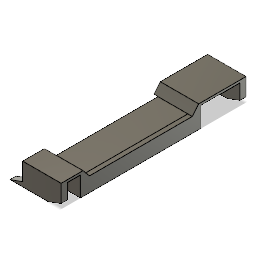
Key v5 (Autodesk Fusion 360 design; units mm, degrees)
Autodesk Fusion 360 part; units mm, degrees
sketch "Sketch1" plane through (0, 0, 0) normal (0, 1, 0) x (1, 0, 0)
  line L0 (15, 72) -> (-15, 72)
  line L1 (-15, 72) -> (-15, -72)
  line L2 (-15, -72) -> (15, -72)
  line L3 (15, -72) -> (15, 72)
  line L4 (15, 72) -> (-15, -72) construction
  line L5 (-15, 72) -> (15, -72) construction
  dimension "d1" = 30
  dimension "d4" = 144
extrude "Extrude1" add sketch "Sketch1" along normal blind 17.5
sketch "Sketch2" plane through (15, 0, 0) normal (1, 0, 0) x (0, 0, -1)
  line L0 (-72, 0) -> (72, 0)
  line L1 (72, 0) -> (72, 17.5)
  line L2 (72, 17.5) -> (-72, 17.5)
  line L3 (-72, 17.5) -> (-72, 0)
  line L4 (-67, 0) -> (-57, 0)
  line L5 (-57, 0) -> (-57, 15.6)
  line L6 (-57, 15.6) -> (-67, 15.6)
  line L7 (-67, 15.6) -> (-67, 0)
  line L8 (67, 0) -> (37, 0)
  line L9 (37, 0) -> (37, 15.6)
  line L10 (37, 15.6) -> (67, 15.6)
  line L11 (67, 15.6) -> (67, 0)
  dimension "d5" = 10
  dimension "d6" = 5
  dimension "d7" = 15.6
  dimension "d8" = 30
  dimension "d9" = 5
  measures "d6" distance of L3 L7
  measures "d7" distance of origin
  measures "d9" distance of L1 L11
extrude "Extrude2" cut sketch "Sketch2" against normal through all contours L0 L4 L5 L6 L7 | L0 L8 L9 L10 L11
sketch "Sketch3" plane through (-15, 0, 0) normal (-1, 0, 0) x (0, 0, 1)
  line L0 (67, 15.6) -> (67, 0)
  line L1 (67, 0) -> (72, 0)
  line L2 (72, 0) -> (72, 17.5)
  line L3 (72, 17.5) -> (-72, 17.5)
  line L4 (-72, 17.5) -> (-72, 0)
  line L5 (-72, 0) -> (-67, 0)
  line L6 (-67, 0) -> (-67, 15.6)
  line L7 (-67, 15.6) -> (-37, 15.6)
  line L8 (-37, 15.6) -> (-37, 0)
  line L9 (-37, 0) -> (57, 0)
  line L10 (57, 0) -> (57, 15.6)
  line L11 (57, 15.6) -> (67, 15.6)
  line L12 (-37, 0) -> (53, 0)
  line L13 (53, 0) -> (53, 7)
  line L14 (53, 7) -> (-37, 7)
  line L15 (-37, 7) -> (-37, 0)
  dimension "d11" = 7
  dimension "d12" = 4
  measures "d11" distance of origin
  measures "d12" distance of L10 L13
extrude "Extrude3" cut sketch "Sketch3" against normal blind 26.5 contours L8 L9 L12 L13 L14 L15
sketch "Sketch4" plane through (-15, 0, 0) normal (-1, 0, 0) x (0, 0, 1)
  line L0 (53, 7) -> (53, 0)
  line L1 (53, 0) -> (57, 0)
  line L2 (57, 0) -> (57, 15.6)
  line L3 (57, 15.6) -> (67, 15.6)
  line L4 (67, 15.6) -> (67, 0)
  line L5 (67, 0) -> (72, 0)
  line L6 (72, 0) -> (72, 17.5)
  line L7 (72, 17.5) -> (-72, 17.5)
  line L8 (-72, 17.5) -> (-72, 0)
  line L9 (-72, 0) -> (-67, 0)
  line L10 (-67, 0) -> (-67, 15.6)
  line L11 (-67, 15.6) -> (-37, 15.6)
  line L12 (-37, 15.6) -> (-37, 7)
  line L13 (-37, 7) -> (53, 7)
  line L14 (-35, 17.5) -> (-30, 11.5)
  line L15 (-30, 11.5) -> (50, 11.5)
  line L16 (50, 11.5) -> (55, 17.5)
  dimension "d15" = 37
  dimension "d16" = 6
  dimension "d17" = 7
  dimension "d18" = 17
  dimension "d19" = 22
  measures "d17" distance of L12
  measures "d19" distance of L6
extrude "Extrude4" cut sketch "Sketch4" against normal through all contours L7 L14 L15 L16
sketch "Sketch5" plane through (-15, 0, 0) normal (-1, 0, 0) x (0, 0, 1)
  line L0 (55, 17.5) -> (50, 11.5)
  line L1 (50, 11.5) -> (-30, 11.5)
  line L2 (-30, 11.5) -> (-35, 17.5)
  line L3 (-35, 17.5) -> (-72, 17.5)
  line L4 (-72, 17.5) -> (-72, 0)
  line L5 (-72, 0) -> (-67, 0)
  line L6 (-67, 0) -> (-67, 15.6)
  line L7 (-67, 15.6) -> (-37, 15.6)
  line L8 (-37, 15.6) -> (-37, 7)
  line L9 (-37, 7) -> (53, 7)
  line L10 (53, 7) -> (53, 0)
  line L11 (53, 0) -> (57, 0)
  line L12 (57, 0) -> (57, 15.6)
  line L13 (57, 15.6) -> (67, 15.6)
  line L14 (67, 15.6) -> (67, 0)
  line L15 (67, 0) -> (72, 0)
  line L16 (72, 0) -> (72, 17.5)
  line L17 (72, 17.5) -> (55, 17.5)
  line L18 (-35, 11.5) -> (55, 11.5)
  line L19 (55, 11.5) -> (55, 8.3)
  line L20 (55, 8.3) -> (-35, 8.3)
  line L21 (-35, 8.3) -> (-35, 11.5)
  dimension "d21" = 5
  dimension "d22" = 3.2
  dimension "d23" = 5
  measures "d21" distance of L21
  measures "d23" distance of L19
extrude "Extrude5" cut sketch "Sketch5" against normal blind 26.5 contours L1 L18 L19 L20 L21
ref_plane "WorkPlane1" through (0, 8.75, 0) normal (0, 0, -1) x (-1, 0, 0)
sketch "Sketch6" plane through (0, 0, -72) normal (0, 0, -1) x (-1, 0, 0)
  line L0 (-15, 0) -> (15, 0)
  line L1 (15, 0) -> (15, 17.5)
  line L2 (15, 17.5) -> (-15, 17.5)
  line L3 (-15, 17.5) -> (-15, 0)
  line L4 (15, 0) -> (25, 0)
  line L5 (25, 0) -> (15, 3.7)
  dimension "d26" = 3.7
  dimension "d27" = 10
  measures "d27" distance of origin
sketch "Sketch7" plane through (0, 0, -72) normal (0, 0, -1) x (-1, 0, 0)
  line L0 (15, 0) -> (-15, 0)
  line L1 (-15, 0) -> (-5, 0)
  line L2 (-15, 0) -> (-15, 17.5)
  line L3 (-5, 0) -> (-15, 3.7)
  line L4 (-15, 0) -> (-15, 3.7)
  dimension "d28" = 10
  dimension "d29" = 3.7
extrude "Extrude6" add sketch "Sketch6" against normal up to surface (5 mm away) contours L1 L4 L5
extrude "Extrude7" cut sketch "Sketch7" against normal up to surface (5 mm away)
mirror "Mirror1" about plane through (0, 8.75, 0) normal (0, 0, -1) of "Extrude6", "Extrude7"
sketch "Sketch8" plane through (0, 0, -72) normal (0, 0, -1) x (-1, 0, 0)
  line L0 (-15, 3.7) -> (-5, 0)
  line L1 (-5, 0) -> (25, 0)
  line L2 (25, 0) -> (15, 3.7)
  line L3 (15, 3.7) -> (15, 17.5)
  line L4 (15, 17.5) -> (-15, 17.5)
  line L5 (-15, 17.5) -> (-15, 3.7)
  circle A0 centre (1.75, 10) radius 2.5
  line L6 (-11.5, 7) -> (15, 7) construction
  line L7 (1.75, 10) -> (1.75, 7) construction
  dimension "d35" = 5
  dimension "d36" = 5
  measures "d35" diameter of A0
  measures "d36" distance of L4 A0
extrude "Extrude8" cut sketch "Sketch8" against normal up to surface (5 mm away) contours A0
sketch "Sketch9" plane through (0, 0, 57) normal (0, 0, 1) x (1, 0, 0)
  line L0 (-15, 15.6) -> (-15, 0)
  line L1 (-15, 0) -> (15, 0)
  line L2 (15, 0) -> (15, 15.6)
  line L3 (15, 15.6) -> (-15, 15.6)
  line L4 (1.25, 12.5) -> (-4.75, 12.5)
  line L5 (-4.75, 12.5) -> (-4.75, 6.5)
  line L6 (-4.75, 6.5) -> (1.25, 6.5)
  line L7 (1.25, 6.5) -> (1.25, 12.5)
  line L8 (1.25, 12.5) -> (-4.75, 6.5) construction
  line L9 (-4.75, 12.5) -> (1.25, 6.5) construction
  line L10 (-15, 8.3) -> (11.5, 8.3) construction
  line L11 (-1.75, 8.3) -> (-1.75, 9.5) construction
  dimension "d39" = 6
  dimension "d40" = 6.5
  measures "d40" distance of L1 L6
extrude "Extrude9" cut sketch "Sketch9" against normal blind 2 contours L4 L5 L6 L7
